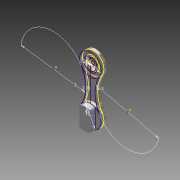
# Autodesk Inventor part: Pneumatic Connector - Side Side
Saved by Autodesk Inventor 2013 (Build 170138000, 138)
## iProperties
Created: 2013-06-08
Part Number: Pneumatic Connector - Side Side
Material: Generic
Document SubType Name: Modeling
Designer: mvarma
Density: 1 g/cm^3
Author: mvarma
Autodesk Inventor part; units mm, degrees
ref_plane "YZ Plane" through (0, 0, 0) normal (1, 0, 0) x (0, 1, 0)
ref_plane "XZ Plane" through (0, 0, 0) normal (0, 1, 0) x (-1, 0, 0)
ref_plane "XY Plane" through (0, 0, 0) normal (0, 0, 1) x (1, 0, 0)
sketch "Sketch6" plane through (0, 0, 0) normal (0, 0, 1) x (1, 0, 0)
  circle A0 centre (0, 0) radius 12.7
  line L0 (0, 12.7) -> (0, 0) construction
  line L1 (0, 0) -> (0, -12.7) construction
  line L2 (-6.35, 10.9985) -> (-6.35, -10.9985)
  line L3 (6.35, 10.9985) -> (6.35, -10.9985)
  line L4 (0, 0) -> (0, 52.324)
  circle A1 centre (0, 52.324) radius 3.175
  circle A2 centre (0, 52.324) radius 7.9375
  circle A3 centre (0, 52.324) radius 12.7
  circle A4 centre (0, 52.324) radius 6.35
  arc A5 (-10.8863, 6.5405) -> (-10.8863, 45.7835) centre (-43.5453, 26.162) ccw
  arc A6 (10.8863, 45.7835) -> (10.8863, 6.5405) centre (43.5453, 26.162) ccw
  dimension "d31" = 25.4
  dimension "d32" = 6.35
  dimension "d46" = 52.324
  dimension "d47" = 6.35
  dimension "d48" = 15.875
  dimension "d49" = 25.4
  dimension "d50" = 12.7
  dimension "d51" = 76.2
  dimension "d52" = 76.2
  constraints: 10 end point, 6 centre point, 6 point on circle, 5 coincident, 3 parallel, 2 tangent, 1 collinear, 1 vertical, 13 other
  measures "d32" distance between parallel lines of L0 L2
  measures "d46" distance of L0.end L4.end
  measures "d47" diameter of A1
  measures "d48" diameter of A2
  measures "d49" diameter of A3
  measures "d50" diameter of A4
  measures "d51" diameter of A5
  measures "d52" diameter of A6
extrude "Extrusion5" add sketch "Sketch6" along normal blind 6.35 contours A0 L2 L3
sketch "Sketch7" plane through (6.35, -10.9985, 0) normal (1, 0, 0) x (0, 0, -1)
  line L0 (0, 0) -> (0, 21.997) projected
  line L1 (0, 21.997) -> (-6.35, 21.997) projected
  line L2 (-6.35, 0) -> (-6.35, 21.997) projected
  line L3 (0, 0) -> (-6.35, 0) projected
  line L4 (-3.175, 21.997) -> (-3.175, 0) construction
  line L5 (-6.35, 10.9985) -> (0, 10.9985) construction
  line L6 (-6.35, 16.4978) -> (0, 16.4978) construction
  line L7 (-6.35, 5.4993) -> (0, 5.4993) construction
  point P0 (-3.175, 16.4978)
  point P1 (-3.175, 5.4993)
  dimension "d35" = 5.4993
  dimension "d36" = 5.4993
  constraints: 8 end point, 5 midpoint, 4 point on line, 3 perpendicular, 1 other
  measures "d35" distance between parallel lines of L5 L6
  measures "d36" distance between parallel lines of L1 L6
hole "Hole3" at (6.35, 5.4993, 3.175) at (6.35, -5.4993, 3.175) direction (-1, 0, 0) diameter 2.6416 end through all thread size "6-32 UNC" class "2B" standard "ANSI Unified Screw Threads"
extrude "Extrusion6" add sketch "Sketch6" against normal blind 3.175 contours A0 L3 | A0 L2 L3 | A0 L2
sketch "Sketch8" plane through (0, 0, -3.175) normal (0, 0, -1) x (-1, 0, 0)
  circle A0 centre (0, 0) radius 12.7 projected
  arc A1 (-10.8863, 6.5405) -> (-10.8863, 45.7835) centre (-43.5453, 26.162) ccw projected
  arc A2 (10.8863, 45.7835) -> (10.8863, 6.5405) centre (43.5453, 26.162) ccw projected
  circle A3 centre (0, 52.324) radius 12.7 projected
  circle A4 centre (0, 52.324) radius 3.175 projected
  circle A5 centre (0, 52.324) radius 6.35 projected
  circle A6 centre (0, 52.324) radius 7.9375 projected
extrude "Extrusion8" add sketch "Sketch8" along normal blind 3.175 contours A0 | A0 A1 A3 A2 | A3
extrude "Extrusion9" add sketch "Sketch8" along normal blind 1.27 contours A6
equation "\"d52\" = d51"
equation "\"d35\" = d36"
body "Solid2"
